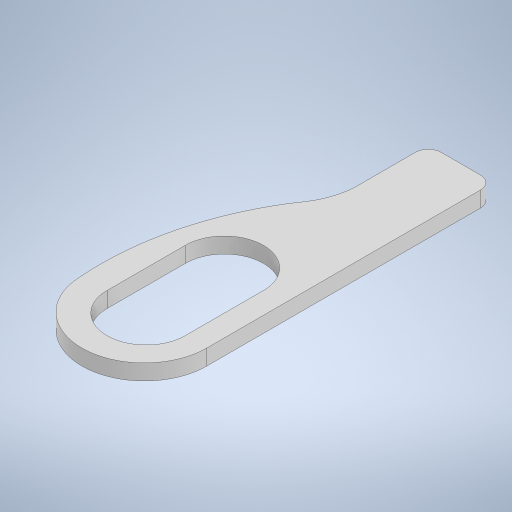
# Autodesk Inventor part: 剪刀握柄
Saved by Autodesk Inventor 2024.2 (Build 282272000, 272)
## iProperties
Created: 2024-05-16
Part Number: 剪刀握柄
Material: 一般
Document SubType Name: Modeling
Designer: User
Density: 1 g/cm^3
Appearance: 預設
Author: User
Autodesk Inventor part; units mm, degrees
ref_plane "YZ Plane" through (0, 0, 0) normal (1, 0, 0) x (0, 1, 0)
ref_plane "XZ Plane" through (0, 0, 0) normal (0, 1, 0) x (-1, 0, 0)
ref_plane "XY Plane" through (0, 0, 0) normal (0, 0, 1) x (1, 0, 0)
sketch "草圖1" plane through (0, 0, 0) normal (0, 1, 0) x (-1, 0, 0)
  line L0 (15, 15) -> (-15, 15)
  line L1 (-15, 15) -> (-15, -15)
  line L2 (-15, -15) -> (15, -15)
  line L3 (15, -15) -> (15, 15)
  line L4 (15, 15) -> (-15, -15) construction
  line L5 (-15, 15) -> (15, -15) construction
  arc A0 (15, 15) -> (-15, 15) centre (0, 15) ccw
  arc A1 (-15, -15) -> (15, -15) centre (0, -15) ccw
  line L6 (0, 15) -> (15, 15)
  line L7 (0, 15) -> (-15, 15)
  arc A2 (24.5849, 17.1216) -> (-23.2433, 15) centre (0.7193, 14.9668) ccw
  line L8 (-23.2433, 15) -> (-23.2433, -90)
  line L9 (25, 15) -> (15, 15)
  line L10 (0, -15) -> (-5, -15)
  line L11 (-18.2433, -95) -> (-3.2433, -95)
  line L12 (-18.2433, -95) -> (-18.2433, -90)
  arc A3 (-23.2433, -90) -> (-18.2433, -95) centre (-18.2433, -90) ccw
  line L13 (-3.2433, -95) -> (-3.2433, -90)
  arc A4 (-3.2433, -95) -> (1.7567, -90) centre (-3.2433, -90) ccw
  arc A5 (7.8049, -50.7012) -> (15, -37.7058) centre (-81.9816, 7.5) ccw
  line L14 (1.7567, -90) -> (1.7567, -66.4736)
  arc A6 (15, -37.7058) -> (24.7552, 15) centre (-81.9816, 7.5) ccw
  arc A7 (7.8049, -50.7012) -> (1.7567, -66.4736) centre (31.6589, -68.8943) ccw
  line L15 (31.6589, -68.8943) -> (3.6477, -58.1529)
  line L16 (0.0146, 7.5) -> (-128.2348, 7.5)
  arc A8 (-23.2433, -81.9361) -> (24.5849, 17.1216) centre (-81.9816, 7.5) ccw
  arc A9 (24.7552, 15) -> (24.5849, 17.1216) centre (-81.9816, 7.5) ccw
  line L17 (-23.2433, -90) -> (1.7567, -90)
  point P0 (0, 0)
  point P1 (24.7552, 15)
  dimension "d0" = 30
  dimension "d1" = 30
  dimension "d2" = 25
  dimension "d5" = 10
  dimension "d6" = 5
  dimension "d9" = 5
  dimension "d10" = 105
  dimension "d11" = 5
  dimension "d12" = 214
  dimension "d16" = 30
  dimension "d17" = 7.5
  dimension "d22" = 25
  constraints: 36 end point, 21 point on circle, 10 centre point, 7 point on line, 6 tangent, 5 horizontal, 3 vertical, 2 coincident, 2 midpoint, 2 parallel, 2 perpendicular, 1 collinear
  measures "d0" distance of L2.end L1.end
  measures "d1" distance of L0.end L1.end
  measures "d2" distance of L6.start L9.start
  measures "d5" distance of L9.start L0.start
  measures "d6" distance of L10.start L10.end
  measures "d9" distance of L11.start L12.end
  measures "d10" distance of L8.start L8.end
  measures "d11" distance of L11.end L13.end
  measures "d12" diameter of A5
  measures "d16" distance of L15.start L15.end
  measures "d17" distance of A2.centre L16.start
  measures "d22" distance of L8.end L14.start
extrude "擠出1" add sketch "草圖1" along normal blind 6 contours L9 A6 A5 A7 A8 L8 L16 L1 A1 L3 | A0 L1 L16 L8 A2 A8 L9 | A8 A7 L14 L17 L8 | L17 L12 A3 | L12 L17 L13 L11 | L13 L17 A4
sketch "草圖4" plane through (18.2433, 0, -95) normal (0, 0, -1) x (-1, 0, 0)
  line L0 (15, 0) -> (15, 6) projected
  line L1 (15, 0) -> (15, 6)
  line L2 (3.2433, 6) -> (33.2433, 6) projected
  line L3 (15, 0) -> (15, 3)
  line L4 (15, 3) -> (15, 1.5)
  line L5 (0, 3) -> (15, 3)
  line L6 (15, 3) -> (15, 4.5)
  line L7 (15, 4.5) -> (0, 4.5)
  line L8 (0, 4.5) -> (0, 3)
  line L9 (0, 3) -> (15, 3)
  point P0 (18.2433, 0)
  dimension "d28" = 1.5
  constraints: 16 end point, 2 midpoint, 2 parallel, 2 point on line, 1 coincident, 1 perpendicular, 1 vertical
  measures "d28" distance of L4.start L6.end
extrude "擠出3" cut sketch "草圖4" against normal blind 10
